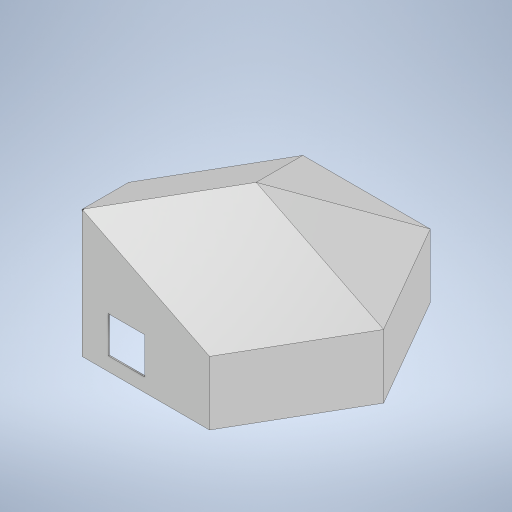
# Autodesk Inventor part: BungaCamp-H13-Hexayurt
Saved by Autodesk Inventor 2023 (Build 270158000, 158)
## iProperties
Created: 2024-07-15
Part Number: BungaCamp-H13-Hexayurt
Material: Generic
Document SubType Name: Modeling
Designer: incep
Density: 1 g/cm^3
Appearance: Default
Author: incep
Autodesk Inventor part; units mm, degrees
sketch "Sketch1" plane through (0, 0, 0) normal (0, 1, 0) x (-1, 0, 0)
  line L0 (-2438.4, 0) -> (-1219.2, 2111.7163)
  line L1 (-1219.2, 2111.7163) -> (1219.2, 2111.7163)
  line L2 (1219.2, 2111.7163) -> (2438.4, 0)
  line L3 (2438.4, 0) -> (1219.2, -2111.7163)
  line L4 (1219.2, -2111.7163) -> (-1219.2, -2111.7163)
  line L5 (-1219.2, -2111.7163) -> (-2438.4, 0)
  line L6 (-2409.0706, 0) -> (-1204.5353, 2086.3163)
  line L7 (-1204.5353, 2086.3163) -> (1204.5353, 2086.3163)
  line L8 (1204.5353, 2086.3163) -> (2409.0706, 0)
  line L9 (2409.0706, 0) -> (1204.5353, -2086.3163)
  line L10 (1204.5353, -2086.3163) -> (-1204.5353, -2086.3163)
  line L11 (-1204.5353, -2086.3163) -> (-2409.0706, 0)
  point P0 (0, 0)
  point P1 (0, 0)
  dimension "d0" = 2438.4
  dimension "d1" = 25.4
  constraints: 24 end point, 1 coincident, 1 horizontal, 18 other
  measures "d0" distance of L3.end L4.end
  measures "d1" distance between parallel lines of L5 L11
extrude "Extrusion1" add sketch "Sketch1" along normal blind 1219.2
sketch "Sketch2" plane through (-1219.2, 0, 2111.7163) normal (0, 0, 1) x (1, 0, 0)
  line L0 (0, 1219.2) -> (2438.4, 1219.2) projected
  line L1 (0, 1219.2) -> (0, 2438.4)
  line L2 (0, 2438.4) -> (2438.4, 1219.2)
  point P0 (1219.2, 0)
  dimension "d4" = 1219.2
  constraints: 4 end point, 1 vertical
  measures "d4" distance of L0.start L1.end
extrude "Extrusion2" add sketch "Sketch2" against normal blind 25.4
sketch "Sketch3" plane through (-2438.4, 0, 0) normal (-0.8660254, 0, 0.5) x (0.5, 0, 0.8660254)
  line L0 (2438.4, 2438.4) -> (2416.403, 2438.4) projected
  line L1 (2438.4, 2438.4) -> (2438.4, 1219.2)
  line L2 (2423.7353, 1219.2) -> (3628.2706, 1219.2) projected
  line L3 (0, 1219.2) -> (2438.4, 1219.2) projected
  line L4 (-1219.2, 1219.2) -> (0, 1219.2) projected
  line L5 (3657.6, 1219.2) -> (2438.4, 2438.4) projected
  line L6 (0, 1219.2) -> (2438.4, 2438.4)
  point P0 (1219.2, 0)
  constraints: 4 end point, 1 point on line, 1 vertical
extrude "Extrusion3" add sketch "Sketch3" against normal blind 25.4
ref_plane "Work Plane1" through (1828.8, 1219.2, 1055.8582) normal (-0.5, 0, 0.8660254) x (-0.8660254, 0, -0.5)
sketch "Sketch5" plane through (1828.8, 1219.2, 1055.8582) normal (-0.5, 0, 0.8660254) x (-0.8660254, 0, -0.5)
  line L0 (0, 0) -> (2111.7163, 0) projected
  line L1 (0, 0) -> (2111.7163, -1219.2)
  line L2 (2111.7163, 0) -> (4223.4327, 0) projected
  line L3 (2111.7163, -1219.2) -> (4223.4327, 0)
  line L4 (0, 0) -> (12.7, 21.997)
  line L5 (12.7, 21.997) -> (2124.4163, -1197.203)
  line L6 (2111.7163, -1219.2) -> (2124.4163, -1197.203)
  line L7 (2111.7163, -1219.2) -> (2099.0163, -1197.203)
  line L8 (4223.4327, 0) -> (4210.7327, 21.997)
  line L9 (4210.7327, 21.997) -> (2099.0163, -1197.203)
  point P0 (2111.7163, 1219.2)
  point P1 (2111.7163, -1189.8706)
  dimension "d9" = 2438.4
  dimension "d10" = 25.4
  dimension "d11" = 25.4
  dimension "d12" = 25.4
  dimension "d13" = 25.4
  constraints: 16 end point, 3 perpendicular, 2 equal length
  measures "d9" distance of L0.start L1.end
  measures "d10" distance of L0.start L4.end
  measures "d11" distance of L1.end L5.end
  measures "d12" distance of L1.end L7.end
  measures "d13" distance of L2.end L8.end
extrude "Extrusion4" add sketch "Sketch5" along normal blind 1219.2 contours L4 L5 L0 | L0 L5 L9 L7 L1 | L6 L5 L9 L2 L3 | L7 L9 L5 L6 | L2 L9 L8
sketch "Sketch6" plane through (-1828.8, 1219.2, -1055.8582) normal (-0.4330127, 0.8660254, -0.25) x (0.75, 0.5, 0.4330127)
  line L0 (2438.4, -1219.2) -> (0, -1219.2) projected
  line L1 (2421.8689, -2416.403) -> (2438.4, -2438.4) projected
  line L2 (2438.4, -1219.2) -> (2438.4, -2438.4)
  line L3 (0, -1219.2) -> (2438.4, -2438.4)
  point P0 (1219.2, 0)
  constraints: 4 end point, 1 vertical
extrude "Extrusion5" add sketch "Sketch6" against normal blind 25.4
sketch "Sketch8" plane through (0, 2438.4, 0) normal (0.4330127, 0.8660254, 0.25) x (0.75, -0.5, 0.4330127)
  line L0 (2438.4, -1219.2) -> (0, -1219.2) projected
  line L1 (0, -2438.4) -> (0, -1219.2) projected
  line L2 (16.4978, -2416.403) -> (0, -2438.4) projected
  line L3 (2438.4, -1219.2) -> (2438.4, 0) projected
  line L4 (0, -2438.4) -> (2438.4, -1219.2)
  point P0 (1219.2, 0)
  constraints: 2 end point
extrude "Extrusion6" add sketch "Sketch8" against normal blind 25.4
sketch "Sketch9" plane through (-1828.8, 1219.2, -1055.8582) normal (-0.4330127, 0.8660254, -0.25) x (0.75, 0.5, 0.4330127)
  line L0 (-609.6, 1219.2) -> (0, 1219.2) projected
  line L1 (2438.4, 0) -> (0, 0) projected
  line L2 (0, 1219.2) -> (2438.4, 0)
  line L3 (0, 1219.2) -> (0, 0) projected
  point P0 (1219.2, 0)
  constraints: 2 end point
extrude "Extrusion7" add sketch "Sketch9" against normal blind 25.4
sketch "Sketch10" plane through (1219.2, 1219.2, 2111.7163) normal (0.4330127, 0.8660254, 0.25) x (0.75, -0.5, 0.4330127)
  line L0 (0, 1219.2) -> (-2438.4, 1219.2) projected
  line L1 (0, 1219.2) -> (0, 2438.4) projected
  line L2 (-2438.4, 1219.2) -> (-3657.6, 2438.4) projected
  line L3 (0, 2438.4) -> (-1828.8, 3657.6) projected
  line L4 (-2438.4, 1219.2) -> (0, 2438.4)
  point P0 (-1219.2, 1219.2)
  constraints: 2 end point
extrude "Extrusion8" add sketch "Sketch10" against normal blind 25.4
ref_plane "Work Plane2" through (2438.4, 1219.2, 0) normal (0.4330127, 0.8660254, -0.25) x (-0.5, 0, -0.8660254)
sketch "Sketch11" plane through (2438.4, 1219.2, 0) normal (0.4330127, 0.8660254, -0.25) x (-0.5, 0, -0.8660254)
  line L0 (0, 0) -> (1219.2, 2438.4) projected
  line L1 (0, 0) -> (2438.4, 0) projected
  line L2 (1219.2, 2438.4) -> (3657.6, 1828.8) projected
  line L3 (2438.4, 0) -> (3657.6, 1828.8) projected
  line L4 (1219.2, 2438.4) -> (2438.4, 0)
  line L5 (1219.2, 2438.4) -> (1222.8662, 2418.236) projected
  line L6 (1219.2, 2438.4) -> (1219.2, 0)
  point P0 (1219.2, 1219.2)
  constraints: 4 end point, 1 midpoint
extrude "Extrusion9" add sketch "Sketch11" against normal blind 25.4 contours L0 L6 L1 | L4 L1 L6
ref_plane "Work Plane3" through (1219.2, 1219.2, -2111.7163) normal (0, -0.8660254, 0.5) x (-0.4472136, 0.4472136, 0.7745967)
sketch "Sketch12" plane through (1219.2, 1219.2, -2111.7163) normal (0, -0.8660254, 0.5) x (-0.4472136, 0.4472136, 0.7745967)
  line L0 (0, 0) -> (1090.4856, 2180.9713) projected
  line L1 (0, 0) -> (2726.2141, 0) projected
  line L2 (1090.4856, 2180.9713) -> (3271.4569, 2453.5927) projected
  line L3 (4907.1853, 272.6214) -> (3271.4569, 2453.5927) projected
  line L4 (4884.2315, 284.0983) -> (4907.1853, 272.6214) projected
  line L5 (4882.5919, 276.7203) -> (4884.2315, 284.0983) projected
  line L6 (4907.1853, 272.6214) -> (4882.5919, 276.7203) projected
  line L7 (2726.2141, 0) -> (4907.1853, 272.6214) projected
  line L8 (2726.2141, 0) -> (1090.4856, 2180.9713) projected
  line L9 (2726.2141, 0) -> (503.3011, 1006.6021)
  point P0 (1635.7284, 545.2428)
  point P1 (1090.4856, 2180.9713)
  constraints: 2 end point, 1 point on line
extrude "Extrusion10" add sketch "Sketch12" along normal blind 25.4 contours L0 L9 L1 | L0 L8 L9
sketch "Sketch13" plane through (-1219.2, 0, 2111.7163) normal (0, 0, 1) x (1, 0, 0)
  line L0 (500, 959.6) -> (1200, 959.6)
  line L1 (1200, 959.6) -> (1200, 259.6)
  line L2 (1200, 259.6) -> (500, 259.6)
  line L3 (500, 259.6) -> (500, 959.6)
  line L4 (2438.4, 0) -> (2438.4, 1219.2) projected
  line L5 (0, 0) -> (0, 2438.4) projected
  point P0 (1219.2, 0)
  point P1 (1200, 609.6)
  point P2 (2438.4, 609.6)
  dimension "d28" = 700
  dimension "d29" = 700
  dimension "d30" = 500
  constraints: 8 end point, 2 midpoint, 2 parallel, 1 horizontal, 1 horizontal alignment, 1 perpendicular
  measures "d28" distance of L0.start L0.end
  measures "d29" distance of L0.end L1.end
  measures "d30" distance between parallel lines of L5 L3
extrude "Extrusion11" cut sketch "Sketch13" against normal up to surface (25.4 mm away)
body "Solid1"
